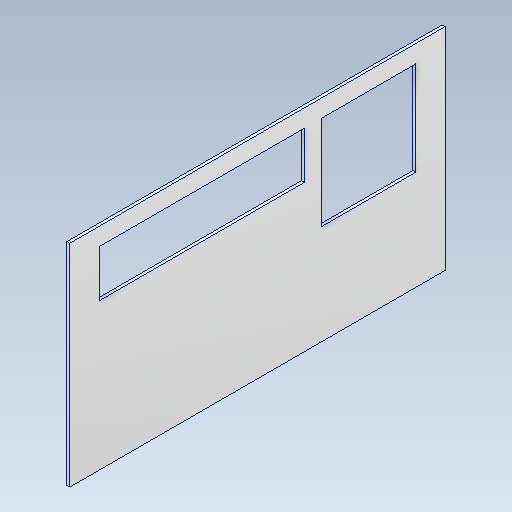
# Autodesk Inventor part: HPStationBase-ver1-1111-2021
Saved by Autodesk Inventor 2021 (Build 250183000, 183)
## iProperties
Created: 2021-03-02
Part Number: HPStationBase-ver1-1111-2021
Material: Aluminum 6061
Document SubType Name: Modeling
Designer: CMurray
Density: 2.7 g/cm^3
Appearance: Aluminum - Flat
Author: CMurray
Autodesk Inventor part; units mm, degrees
ref_plane "YZ Plane" through (0, 0, 0) normal (1, 0, 0) x (0, 1, 0)
ref_plane "XZ Plane" through (0, 0, 0) normal (0, 1, 0) x (-1, 0, 0)
ref_plane "XY Plane" through (0, 0, 0) normal (0, 0, 1) x (1, 0, 0)
sketch "Sketch1" plane through (0, 0, 0) normal (1, 0, 0) x (0, 1, 0)
  line L0 (0, 0) -> (914.4, 0)
  line L1 (914.4, 0) -> (914.4, -1625.6)
  line L2 (914.4, -1625.6) -> (0, -1625.6)
  line L3 (0, -1625.6) -> (0, 0)
  dimension "d0" = 1625.6
  dimension "d1" = 914.4
  constraints: 8 end point, 2 parallel, 1 horizontal, 1 perpendicular
  measures "d0" distance between parallel lines of L2 L0
  measures "d1" distance between parallel lines of L3 L1
extrude "Extrusion1" add sketch "Sketch1" along normal blind 12.7
sketch "Sketch3" plane through (12.7, 0, 0) normal (1, 0, 0) x (0, 0, -1)
  line L0 (0, 0) -> (1625.6, 0) projected
  line L1 (1625.6, 0) -> (1625.6, 914.4) projected
  line L2 (127, 838.2) -> (1016, 838.2)
  line L3 (1016, 838.2) -> (1016, 635)
  line L4 (1016, 635) -> (127, 635)
  line L5 (127, 635) -> (127, 838.2)
  line L6 (0, 914.4) -> (0, 0) projected
  line L7 (1092.2, 838.2) -> (1498.6, 838.2)
  line L8 (1498.6, 838.2) -> (1498.6, 431.8)
  line L9 (1498.6, 431.8) -> (1092.2, 431.8)
  line L10 (1092.2, 431.8) -> (1092.2, 838.2)
  line L11 (1625.6, 914.4) -> (0, 914.4) projected
  dimension "d12" = 889
  dimension "d13" = 203.2
  dimension "d14" = 127
  dimension "d15" = 406.4
  dimension "d16" = 406.4
  dimension "d17" = 76.2
  dimension "d18" = 76.2
  dimension "d19" = 127
  constraints: 16 end point, 4 parallel, 2 horizontal, 2 perpendicular
  measures "d12" distance between parallel lines of L3 L5
  measures "d13" distance between parallel lines of L4 L2
  measures "d14" distance between parallel lines of L5 L6
  measures "d15" distance between parallel lines of L8 L10
  measures "d16" distance between parallel lines of L9 L7
  measures "d17" distance between parallel lines of L7 L11
  measures "d18" distance between parallel lines of L2 L11
  measures "d19" distance between parallel lines of L8 L1
extrude "Extrusion3" cut sketch "Sketch3" against normal blind 127 contours L2 L3 L4 L5 | L7 L8 L9 L10
body "Solid1"
